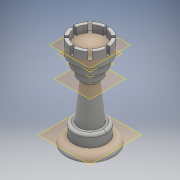
# Autodesk Inventor part: Chess Tower
Saved by Autodesk Inventor 2016 (Build 200138000, 138)
## iProperties
Created: 2019-12-01
Part Number: Chess Tower
Material: Generic
Document SubType Name: Modeling
Designer: wilbi
Density: 1 g/cm^3
Appearance: Default
Author: wilbi
Autodesk Inventor part; units mm, degrees
ref_plane "YZ Plane" through (0, 0, 0) normal (1, 0, 0) x (0, 1, 0)
ref_plane "XZ Plane" through (0, 0, 0) normal (0, 1, 0) x (-1, 0, 0)
ref_plane "XY Plane" through (0, 0, 0) normal (0, 0, 1) x (1, 0, 0)
sketch "Sketch1" plane through (0, 0, 0) normal (0, 0, 1) x (1, 0, 0)
  circle A0 centre (0, 0) radius 16
  dimension "d0" = 32
  constraints: 1 centre point, 1 coincident
  measures "d0" diameter of A0
extrude "Extrusion1" add sketch "Sketch1" along normal blind 5
ref_plane "Work Plane1" through (0, 0, 5) normal (0, 0, 1) x (1, 0, 0)
sketch "Sketch2" plane through (0, 0, 5) normal (0, 0, 1) x (1, 0, 0)
  circle A0 centre (0, 0) radius 11
  dimension "d4" = 22
  constraints: 1 centre point, 1 coincident
  measures "d4" diameter of A0
extrude "Extrusion2" add sketch "Sketch2" along normal blind 8
fillet "Fillet1" radius 5 1 edges at (-16, 0, 5)
sketch "Sketch3" plane through (0, 0, 13) normal (0, 0, 1) x (1, 0, 0)
  point P0 (0, 0)
sketch "Sketch4" plane through (0, 0, 13) normal (0, 0, 1) x (1, 0, 0)
  point P0 (0, 0)
sketch "Sketch5" plane through (0, 0, 13) normal (0, 0, 1) x (1, 0, 0)
  circle A0 centre (0, 0) radius 7.5
  dimension "d8" = 15
  constraints: 1 centre point, 1 coincident
  measures "d8" diameter of A0
ref_plane "Work Plane2" through (0, 0, 38) normal (0, 0, 1) x (1, 0, 0)
sketch "Sketch6" plane through (0, 0, 38) normal (0, 0, 1) x (1, 0, 0)
  circle A0 centre (0, 0) radius 5
  dimension "d10" = 10
  constraints: 1 centre point, 1 coincident
  measures "d10" diameter of A0
loft "Loft1" add profiles "Sketch6", "Sketch5"
ref_plane "Work Plane3" through (0, 0, 41) normal (0, 0, 1) x (1, 0, 0)
sketch "Sketch7" plane through (0, 0, 41) normal (0, 0, 1) x (1, 0, 0)
  circle A0 centre (0, 0) radius 7.5
  dimension "d16" = 15
  constraints: 1 centre point, 1 coincident
  measures "d16" diameter of A0
loft "Loft2" add profiles "Sketch7" section 1 edges at (-5, 0, 38)
sketch "Sketch8" plane through (0, 0, 41) normal (0, 0, 1) x (1, 0, 0)
  circle A0 centre (0, 0) radius 7.5
  constraints: 1 centre point, 1 coincident
extrude "Extrusion3" add sketch "Sketch8" along normal blind 3
ref_plane "Work Plane4" through (0, 0, 47) normal (0, 0, 1) x (1, 0, 0)
sketch "Sketch9" plane through (0, 0, 47) normal (0, 0, 1) x (1, 0, 0)
  circle A0 centre (0, 0) radius 10
  dimension "d24" = 20
  constraints: 1 centre point, 1 coincident
  measures "d24" diameter of A0
loft "Loft3" add profiles "Sketch9" section 2 edges at (-7.5, 0, 44)
sketch "Sketch10" plane through (0, 0, 47) normal (0, 0, 1) x (1, 0, 0)
  circle A0 centre (0, 0) radius 10
  dimension "d29" = 20
  constraints: 1 centre point, 1 coincident
  measures "d29" diameter of A0
extrude "Extrusion4" add sketch "Sketch10" along normal blind 3
ref_plane "Work Plane5" through (0, 0, 53) normal (0, 0, 1) x (1, 0, 0)
sketch "Sketch11" plane through (0, 0, 53) normal (0, 0, 1) x (1, 0, 0)
  circle A0 centre (0, 0) radius 12.5
  dimension "d33" = 25
  constraints: 1 centre point, 1 coincident
  measures "d33" diameter of A0
loft "Loft4" add profiles "Sketch11" section 2 edges at (-10, 0, 50)
sketch "Sketch16" plane through (0, 0, 53) normal (0, 0, 1) x (1, 0, 0)
  circle A0 centre (0, 0) radius 12.5
  dimension "d71" = 25
  constraints: 1 centre point, 1 coincident
  measures "d71" diameter of A0
extrude "Extrusion7" add sketch "Sketch16" along normal blind 5
ref_plane "Work Plane7" through (0, 0, 58) normal (0, 0, 1) x (1, 0, 0)
sketch "Sketch17" plane through (0, 0, 58) normal (0, 0, 1) x (1, 0, 0)
  point P0 (0, 0)
sketch "Sketch18" plane through (0, 0, 58) normal (0, 0, 1) x (1, 0, 0)
  line L0 (-1, -1) -> (0.3304, -1) construction
  line L1 (-1, 1) -> (1.4692, 1) construction
  line L2 (8.1317, 9.5459) -> (6.5185, 7.9328)
  line L3 (9.5459, 8.1317) -> (7.9355, 6.5212)
  line L4 (12.4599, 1) -> (10.2286, 1)
  line L5 (12.4599, -1) -> (10.2286, -1)
  line L6 (7.9355, -6.5212) -> (9.5176, -8.1034)
  line L7 (6.5185, -7.9328) -> (8.1034, -9.5176)
  line L8 (1, -12.4599) -> (1, -10.2038)
  line L9 (-1, -12.4599) -> (-1, -10.1984)
  line L10 (-6.4937, -7.908) -> (-8.1317, -9.5459)
  line L11 (-7.9053, -6.4911) -> (-9.5459, -8.1317)
  line L12 (-10.1736, -1) -> (-12.4599, -1)
  line L13 (-10.1736, 1) -> (-12.4599, 1)
  line L14 (-9.5176, 8.1034) -> (-7.9053, 6.4911)
  line L15 (-8.1034, 9.5176) -> (-6.4937, 7.908)
  line L16 (-1, 10.1984) -> (-1, 12.4599)
  line L17 (1, 10.2038) -> (1, 12.4599)
  arc A0 (-6.4937, -7.908) -> (-1, -10.1984) centre (0.0275, 0) ccw
  arc A1 (-10.1736, -1) -> (-7.9053, -6.4911) centre (0.0275, 0) ccw
  arc A2 (-12.4599, -1) -> (-9.5176, -8.1034) centre (0, 0) ccw
  arc A3 (-8.1034, -9.5176) -> (-1, -12.4599) centre (0, 0) ccw
  arc A4 (-7.9053, 6.4911) -> (-10.1736, 1) centre (0.0275, 0) ccw
  arc A5 (-9.5176, 8.1034) -> (-12.4599, 1) centre (0, 0) ccw
  arc A6 (-1, 12.4599) -> (-8.1034, 9.5176) centre (0, 0) ccw
  arc A7 (-1, 10.1984) -> (-6.4937, 7.908) centre (0.0275, 0) ccw
  arc A8 (8.1034, 9.5176) -> (1, 12.4599) centre (0, 0) ccw
  arc A9 (6.5185, 7.9328) -> (1, 10.2038) centre (0.0275, 0) ccw
  arc A10 (10.2286, 1) -> (7.9355, 6.5212) centre (0.0275, 0) ccw
  arc A11 (12.4599, 1) -> (9.5176, 8.1034) centre (0, 0) ccw
  arc A12 (1, -10.2038) -> (6.5185, -7.9328) centre (0.0275, 0) ccw
  arc A13 (7.9355, -6.5212) -> (10.2286, -1) centre (0.0275, 0) ccw
  arc A14 (1, -12.4599) -> (8.1034, -9.5176) centre (0, 0) ccw
  arc A15 (9.5176, -8.1034) -> (12.4599, -1) centre (0, 0) ccw
  point P0 (0, 0)
  constraints: 36 end point, 32 point on circle, 16 centre point, 4 point on line, 2 horizontal, 1 coincident
extrude "Extrusion8" add sketch "Sketch18" along normal blind 5
fillet "Fillet2" radius 2 1 edges at (-11, 0, 13) curvature continuous yes
sketch "Sketch19" plane through (0, 0, 0) normal (0, 0, -1) x (-1, 0, 0)
  point P0 (0, 0)
body "Solid1"
